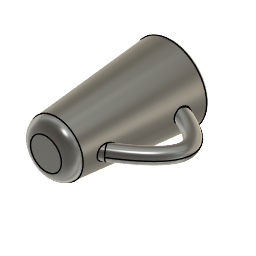
lab4 (Autodesk Fusion 360 design; units mm, degrees)
part number: 2026-03-23-18-16-22-813
Autodesk Fusion 360 part; units mm, degrees
sketch "Sketch1" plane through (0, 0, 0) normal (0, 0, 1) x (1, 0, 0)
  line L0 (0, 0) -> (14.9204, 0)
  line L1 (25.8785, 10.0413) -> (35.4797, 119.7839)
  line L2 (14.9204, 0) -> (-95, 0) construction
  line L3 (21.8559, 21.4312) -> (30.4988, 120.2197)
  line L4 (0, 5) -> (3.9244, 5)
  arc A0 (3.9244, 5) -> (21.8559, 21.4312) centre (3.9244, 23) ccw
  arc A1 (14.9204, 0) -> (25.8785, 10.0413) centre (14.9204, 11) ccw
  arc A2 (35.4797, 119.7839) -> (30.4988, 120.2197) centre (32.9892, 120.0018) ccw
  line L5 (0, 5) -> (0, 0)
  line L6 (0, 170) -> (0, 0) construction
  spline S0 degree 5 poles (33.5808, 98.0791) (36.083, 97.052) (40.8513, 94.9695) (47.2957, 91.7608) (54.4487, 87.3099) (60.8347, 81.44) (64.463, 75.2395) (65.1493, 68.6862) (62.8676, 61.777) (57.8071, 54.5347) (50.2101, 46.9883) (42.2852, 40.7297) (35.3708, 35.9193) (30.3369, 32.6616) (27.7139, 31.02) knots 0 0 0 0 0 0 0.1 0.2 0.3 0.4 0.5 0.6 0.7 0.8 0.9 1 1 1 1 1 1
  point P0 (64.5093, 70.8254)
  dimension "d2" = 95
  dimension "d7" = 11
  dimension "d8" = 2.5
  dimension "d9" = 32.9892
  dimension "d10" = 14.9204
  dimension "d11" = 21.8559
  constraint coincident L0.start L5.end
  constraint horizontal L0
  constraint horizontal L2
  constraint tangent L3 A0
  constraint tangent L4 A0
  constraint tangent L1 A1
  constraint tangent L2 A1
  constraint perpendicular L2 L5
  constraint perpendicular L2 L6
  constraint coincident L1 S0.start
  constraint coincident L1 S0.end
  measures "d2" angle of L1 L2
  measures "d7" radius of A1
  measures "d8" radius of A2
  measures "d9" distance of A2.centre L6
  measures "d10" distance of A1.centre L6
  measures "d11" distance of L3.start L6
revolve "Revolve1" add sketch "Sketch1" angle 360 about axis through (0, 170, 0) along (0, -1, 0) contours L0 L1 L3 L4 A0 A1 A2 L5
ref_plane "WorkPlane1" through (33.5808, 98.0791, 0) normal (0.925094, -0.379738, 0) x (-0.379738, -0.925094, 0)
sketch "Sketch4" plane through (33.5808, 98.0791, 0) normal (0.925094, -0.379738, 0) x (-0.379738, -0.925094, 0)
  circle A0 centre (0, 0) radius 6.8184
  constraint coincident A0.centre origin
sweep "Sweep1" add profiles "Sketch4" path "Sketch1" along S0 section 1
extrude "Extrude1" add 1 faces at (28.7787, 29.3185, 1.7135) along direction (-0.847676, -0.530514, 0) blind 6
extrude "Extrude2" add 1 faces at (34.3964, 100.0661, 1.1133) along direction (-0.925094, 0.379738, 0) blind 4
